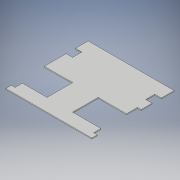
# Autodesk Inventor part: ElectricalBoard.ver2-1111-2020
Saved by Autodesk Inventor 2018 (Build 220112000, 112)
## iProperties
Created: 2020-01-21
Part Number: ElectricalBoard.ver2-1111-2020
Material: Generic
Document SubType Name: Modeling
Designer: JMHal
Density: 1 g/cm^3
Appearance: Default
Author: JMHal
Autodesk Inventor part; units mm, degrees
ref_plane "YZ Plane" through (0, 0, 0) normal (1, 0, 0) x (0, 1, 0)
ref_plane "XZ Plane" through (0, 0, 0) normal (0, 1, 0) x (-1, 0, 0)
ref_plane "XY Plane" through (0, 0, 0) normal (0, 0, 1) x (1, 0, 0)
sketch "Sketch1" plane through (0, 0, 0) normal (0, 1, 0) x (-1, 0, 0)
  line L0 (0, 0) -> (596.9, 0)
  line L1 (596.9, 0) -> (596.9, -571.5)
  line L2 (596.9, -571.5) -> (0, -571.5)
  line L3 (0, -571.5) -> (0, 0)
  line L4 (596.9, 0) -> (0, 0)
  line L5 (0, 0) -> (0, -38.1)
  line L6 (0, -38.1) -> (596.9, -38.1)
  line L7 (596.9, -38.1) -> (596.9, 0)
  line L8 (25.4, -38.1) -> (571.5, -38.1)
  line L9 (571.5, -38.1) -> (571.5, -88.9)
  line L10 (571.5, -88.9) -> (25.4, -88.9)
  line L11 (25.4, -88.9) -> (25.4, -38.1)
  line L12 (400.05, -88.9) -> (222.25, -88.9)
  line L13 (222.25, -88.9) -> (222.25, -266.7)
  line L14 (222.25, -266.7) -> (400.05, -266.7)
  line L15 (400.05, -266.7) -> (400.05, -88.9)
  line L16 (596.9, -266.7) -> (0, -266.7)
  line L17 (0, -266.7) -> (0, -342.9)
  line L18 (0, -342.9) -> (596.9, -342.9)
  line L19 (596.9, -342.9) -> (596.9, -266.7)
  line L20 (568.9457, -342.9) -> (52.0133, -342.9)
  line L21 (52.0133, -419.1) -> (568.9457, -419.1)
  line L22 (596.9, -419.1) -> (0, -419.1)
  line L23 (0, -419.1) -> (0, -571.5)
  line L24 (0, -571.5) -> (596.9, -571.5)
  line L25 (596.9, -571.5) -> (596.9, -419.1)
  line L26 (571.5, -266.7) -> (25.4, -266.7)
  line L27 (25.4, -266.7) -> (25.4, -342.9)
  line L28 (25.4, -342.9) -> (571.5, -342.9)
  line L29 (571.5, -342.9) -> (571.5, -266.7)
  line L30 (552.45, -419.1) -> (44.45, -419.1)
  line L31 (44.45, -419.1) -> (44.45, -508)
  line L32 (44.45, -508) -> (552.45, -508)
  line L33 (552.45, -508) -> (552.45, -419.1)
  line L34 (596.9, -571.5) -> (0, -571.5)
  line L35 (0, -571.5) -> (0, -482.6)
  line L36 (0, -482.6) -> (596.9, -482.6)
  line L37 (596.9, -482.6) -> (596.9, -571.5)
  dimension "d0" = 596.9
  dimension "d1" = 571.5
  dimension "d2" = 38.1
  dimension "d3" = 50.8
  dimension "d4" = 177.8
  dimension "d6" = 76.2
  dimension "d7" = 76.2
  dimension "d8" = 88.9
  dimension "d9" = 88.9
  dimension "d10" = 44.45
  dimension "d11" = 44.45
  dimension "d12" = 25.4
  dimension "d13" = 25.4
  dimension "d14" = 177.8
  dimension "d15" = 196.85
  dimension "d16" = 25.4
  dimension "d17" = 25.4
  constraints: 76 end point, 19 parallel, 13 point on line, 10 horizontal, 9 perpendicular
  measures "d0" distance of L1.end L2.end
  measures "d1" distance of L0.end L1.end
  measures "d2" distance between parallel lines of L0 L8
  measures "d3" distance between parallel lines of L12 L6
  measures "d4" distance between parallel lines of L16 L10
  measures "d6" distance between parallel lines of L21 L20
  measures "d7" distance between parallel lines of L20 L14
  measures "d8" distance of L32.end L30.start
  measures "d9" distance between parallel lines of L2 L36
  measures "d10" distance between parallel lines of L31 L3
  measures "d11" distance between parallel lines of L1 L33
  measures "d12" distance between parallel lines of L1 L29
  measures "d13" distance between parallel lines of L3 L27
  measures "d14" distance between parallel lines of L15 L13
  measures "d15" distance between parallel lines of L1 L15
  measures "d16" distance between parallel lines of L3 L11
  measures "d17" distance between parallel lines of L1 L9
extrude "Extrusion1" add sketch "Sketch1" along normal blind 6.35 contours L0 L1 L6 L3 | L6 L9 L10 L11 | L1 L18 L29 L16 | L18 L1 L22 L21 L3 | L16 L14 L29 L18 L27 | L13 L10 L15 L14 | L36 L31 L32 L33 L1 L2 L3 | L22 L21 L33 L36 L31 | L36 L33 L32 L31
body "Solid1"
